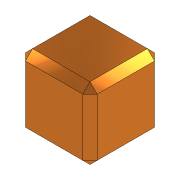
# Autodesk Inventor part: ElementaryCube
Saved by Autodesk Inventor 2021 (Build 250183000, 183)
## iProperties
Created: 2021-04-01
Part Number: ElementaryCube
Material: Gold
Document SubType Name: Modeling
Designer: Tran Duc Viet
Mass: 2280.62 g
Surface Area: 131.673 cm^2
Volume: 118.167 cm^3
Density: 19.3 g/cm^3
Appearance: Metal 1600F Hot
Author: Tran Duc Viet
Autodesk Inventor part; units mm, degrees
ref_plane "YZ Plane" through (0, 0, 0) normal (1, 0, 0) x (0, 1, 0)
ref_plane "XZ Plane" through (0, 0, 0) normal (0, 1, 0) x (-1, 0, 0)
ref_plane "XY Plane" through (0, 0, 0) normal (0, 0, 1) x (1, 0, 0)
sketch "Sketch1" plane through (0, 0, 0) normal (0, 1, 0) x (-1, 0, 0)
  line L0 (25, 25) -> (-25, 25)
  line L1 (-25, 25) -> (-25, -25)
  line L2 (-25, -25) -> (25, -25)
  line L3 (25, -25) -> (25, 25)
  line L4 (25, 25) -> (-25, -25) construction
  line L5 (-25, 25) -> (25, -25) construction
  point P0 (0, 0)
  dimension "d0" = 50
  dimension "d1" = 50
  constraints: 12 end point, 2 midpoint, 2 parallel, 1 horizontal, 1 perpendicular
  measures "d0" distance of L2.end L1.end
  measures "d1" distance of L1.end L0.end
extrude "Extrusion1" add sketch "Sketch1" along normal mid plane 50
chamfer "Chamfer1" distance 5 angle 45 12 edges at (25, 0, -25) (0, 25, -25) (-25, 0, -25) (-25, 25, 0) (-25, 0, 25) (25, 0, 25) (0, -25, -25) (-25, -25, 0) (0, -25, 25) (25, -25, 0) (25, 25, 0) (0, 25, 25)
body "Solid1"
